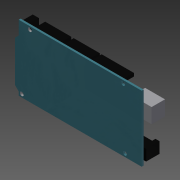
# Autodesk Inventor part: ArduinoMega
Saved by Autodesk Inventor 2014 SP1 (Build 180222100, 222)
## iProperties
Created: 2014-02-09
Part Number: ArduinoMega
Material: Generic
Document SubType Name: Modeling
Designer: Jack
Density: 1 g/cm^3
Appearance: Default
Author: Jack
Autodesk Inventor part; units mm, degrees
ref_plane "YZ Plane" through (0, 0, 0) normal (1, 0, 0) x (0, 1, 0)
ref_plane "XZ Plane" through (0, 0, 0) normal (0, 1, 0) x (-1, 0, 0)
ref_plane "XY Plane" through (0, 0, 0) normal (0, 0, 1) x (1, 0, 0)
sketch "Sketch1" plane through (0, 0, 0) normal (0, 1, 0) x (-1, 0, 0)
  line L0 (0, 0) -> (99, 0)
  line L1 (99, 0) -> (99, 3)
  line L2 (99, 3) -> (102, 6)
  line L3 (102, 6) -> (102, 39)
  line L4 (102, 39) -> (99, 42)
  line L5 (99, 42) -> (99, 53)
  line L6 (99, 53) -> (0, 53)
  line L7 (0, 53) -> (0, 0)
  dimension "d0" = 99
  dimension "d1" = 3
  dimension "d2" = 135
  dimension "d3" = 33
  dimension "d4" = 3
  dimension "d5" = 3
  dimension "d6" = 53
  constraints: 16 end point, 4 perpendicular, 2 parallel, 1 horizontal
  measures "d0" distance of L0.start L0.end
  measures "d1" distance of L0.end L1.end
  measures "d2" angle of L1 L2
  measures "d3" distance of L2.end L3.end
  measures "d4" distance between parallel lines of L1 L3
  measures "d5" distance between parallel lines of L3 L5
  measures "d6" distance between parallel lines of L0 L6
extrude "Extrusion1" add sketch "Sketch1" along normal blind 1.6
sketch "Sketch2" plane through (0, 1.6, 0) normal (0, 1, 0) x (1, 0, 0)
  line L0 (0, 0) -> (-99, 0) projected
  line L1 (0, -53) -> (0, 0) projected
  line L2 (2, -3.8) -> (-12, -3.8)
  line L3 (-12, -3.8) -> (-12, -12.6)
  line L4 (-12, -12.6) -> (2, -12.6)
  line L5 (2, -12.6) -> (2, -3.8)
  dimension "d9" = 8.8
  dimension "d10" = 2
  dimension "d11" = 3.8
  dimension "d12" = 14
  constraints: 8 end point, 2 parallel, 1 horizontal, 1 perpendicular
  measures "d9" distance of L2.end L3.end
  measures "d10" distance between parallel lines of L1 L5
  measures "d11" distance between parallel lines of L0 L2
  measures "d12" distance of L2.start L2.end
extrude "Extrusion2" add sketch "Sketch2" along normal blind 10.8
sketch "Sketch3" plane through (-12, 1.6, 3.8) normal (-1, 0, 0) x (0, 0, 1)
  line L0 (8.8, 0) -> (0, 0) projected
  line L1 (8.8, 0) -> (8.8, 10.8) projected
  line L2 (0, 10.8) -> (8.8, 10.8) projected
  line L3 (0, 0) -> (0, 10.8) projected
  arc A0 (8.8, 6.4) -> (0, 6.4) centre (4.4, 6.4) ccw
  point P0 (-3.8, -1.6)
  constraints: 3 tangent, 2 point on circle, 2 point on line, 1 centre point
extrude "Extrusion3" cut sketch "Sketch3" against normal blind 10.7 contours A0 L2 L1 | L3 L2 A0
sketch "Sketch4" plane through (0, 1.6, 0) normal (0, 1, 0) x (1, 0, 0)
  line L0 (-99, -53) -> (0, -53) projected
  line L1 (0, -53) -> (0, -12.6) projected
  line L2 (-9.6, -32) -> (6.4, -32)
  line L3 (6.4, -32) -> (6.4, -44)
  line L4 (6.4, -44) -> (-9.6, -44)
  line L5 (-9.6, -44) -> (-9.6, -32)
  dimension "d17" = 16
  dimension "d18" = 12
  dimension "d19" = 6.4
  dimension "d20" = 9
  constraints: 8 end point, 2 parallel, 1 horizontal, 1 perpendicular
  measures "d17" distance of L2.start L2.end
  measures "d18" distance of L4.end L2.start
  measures "d19" distance between parallel lines of L1 L3
  measures "d20" distance between parallel lines of L0 L4
extrude "Extrusion4" add sketch "Sketch4" along normal blind 10.8
sketch "Sketch5" plane through (0, 1.6, 0) normal (0, 1, 0) x (1, 0, 0)
  line L0 (0, -3.8) -> (0, 0) projected
  line L1 (0, 0) -> (-99, 0) projected
  line L2 (-26, -3.5) -> (-47, -3.5)
  line L3 (-47, -3.5) -> (-47, -1)
  line L4 (-47, -1) -> (-26, -1)
  line L5 (-26, -1) -> (-26, -3.5)
  line L6 (-48.8, -3.5) -> (-69.8, -3.5)
  line L7 (-69.8, -3.5) -> (-69.8, -1)
  line L8 (-69.8, -1) -> (-48.8, -1)
  line L9 (-48.8, -1) -> (-48.8, -3.5)
  line L10 (-71.6, -3.5) -> (-92.6, -3.5)
  line L11 (-92.6, -3.5) -> (-92.6, -1)
  line L12 (-92.6, -1) -> (-71.6, -1)
  line L13 (-71.6, -1) -> (-71.6, -3.5)
  dimension "d23" = 21
  dimension "d24" = 2.5
  dimension "d25" = 26
  dimension "d26" = 1
  dimension "d29" = 22.8
  constraints: 24 end point, 2 horizontal, 2 parallel, 1 perpendicular, 16 other
  measures "d23" distance of L2.start L2.end
  measures "d24" distance of L2.end L3.end
  measures "d25" distance between parallel lines of L0 L5
  measures "d26" distance between parallel lines of L1 L4
  measures "d29" distance of L2.start L6.start
extrude "Extrusion5" add sketch "Sketch5" along normal blind 8.7
sketch "Sketch6" plane through (0, 1.6, 0) normal (0, 1, 0) x (1, 0, 0)
  line L0 (0, 0) -> (-99, 0) projected
  line L1 (-102, -6) -> (-102, -39) projected
  line L2 (-98, -6) -> (-93, -6)
  line L3 (-93, -6) -> (-93, -52)
  line L4 (-93, -52) -> (-98, -52)
  line L5 (-98, -52) -> (-98, -6)
  dimension "d36" = 46
  dimension "d37" = 5
  dimension "d38" = 4
  dimension "d39" = 6
  constraints: 8 end point, 2 parallel, 1 horizontal, 1 perpendicular
  measures "d36" distance of L2.end L3.end
  measures "d37" distance of L2.start L2.end
  measures "d38" distance between parallel lines of L1 L5
  measures "d39" distance between parallel lines of L0 L2
extrude "Extrusion6" add sketch "Sketch6" along normal blind 8.7
sketch "Sketch7" plane through (0, 1.6, 0) normal (0, 1, 0) x (1, 0, 0)
  line L0 (-99, -42) -> (-99, -53) projected
  line L1 (-99, -53) -> (0, -53) projected
  line L2 (-88, -49.5) -> (-67, -49.5)
  line L3 (-67, -49.5) -> (-67, -52)
  line L4 (-67, -52) -> (-88, -52)
  line L5 (-88, -52) -> (-88, -49.5)
  line L6 (-65, -49.5) -> (-44, -49.5)
  line L7 (-44, -49.5) -> (-44, -52)
  line L8 (-44, -52) -> (-65, -52)
  line L9 (-65, -52) -> (-65, -49.5)
  line L10 (-42.5, -49.5) -> (-16.5, -49.5)
  line L11 (-16.5, -49.5) -> (-16.5, -52)
  line L12 (-16.5, -52) -> (-42.5, -52)
  line L13 (-42.5, -52) -> (-42.5, -49.5)
  dimension "d42" = 21
  dimension "d43" = 2.5
  dimension "d44" = 1
  dimension "d45" = 11
  dimension "d48" = 23
  dimension "d54" = 26
  dimension "d55" = 1
  dimension "d56" = 1.5
  constraints: 24 end point, 5 parallel, 3 horizontal, 2 perpendicular, 8 other
  measures "d42" distance of L3.end L4.end
  measures "d43" distance of L2.end L3.end
  measures "d44" distance between parallel lines of L1 L4
  measures "d45" distance between parallel lines of L0 L5
  measures "d48" distance of L2.start L6.start
  measures "d54" distance of L10.start L10.end
  measures "d55" distance between parallel lines of L1 L12
  measures "d56" distance between parallel lines of L7 L13
extrude "Extrusion7" add sketch "Sketch7" along normal blind 8.7
hole "Hole1" at (-96.5, 1.6, 2.5) direction (0, -1, 0) diameter 3 end through all
hole "Hole2" at (-90, 1.6, 50.5) direction (0, -1, 0) diameter 3 end through all
hole "Hole3" at (-13.5, 1.6, 2.5) direction (0, -1, 0) diameter 3 end through all
hole "Hole4" at (-15, 1.6, 50.447) direction (0, -1, 0) diameter 3 end through all
body "Solid1"
